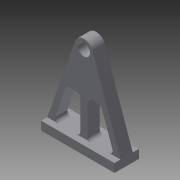
# Autodesk Inventor part: Y_axis_shaft_end_support
Saved by Autodesk Inventor 2013 (Build 170138000, 138)
## iProperties
Created: 2013-09-20
Part Number: Y_axis_shaft_end_support
Material: Aluminum 6061
Document SubType Name: Modeling
Designer: Ian
Density: 2.71 g/cm^3
Mass: 125.761 g
Surface Area: 152.318 cm^2
Volume: 46.4061 cm^3
d0: 3.500 in
d2: 0.500 in
d3: 0.750 in
d5: 1.500 in
d6: 90.00 deg
d7: 0.350 in
d14: 0.250 in
d16: 0.300 in
d17: 70.71 deg
d18: 0.150 in
d19: 0.300 in
d20: 0.300 in
d21: 0.300 in
d22: 0.150 in
d23: 0.150 in
d24: 0.500 in
d25: 0.150 in
d26: 0.500 in
d27: 0.00 deg
d28: 0.250 in
d29: 0.00 deg
Author: Ian
Autodesk Inventor part; units mm, degrees
ref_plane "YZ Plane" through (0, 0, 0) normal (1, 0, 0) x (0, 1, 0)
ref_plane "XZ Plane" through (0, 0, 0) normal (0, 1, 0) x (-1, 0, 0)
ref_plane "XY Plane" through (0, 0, 0) normal (0, 0, 1) x (1, 0, 0)
sketch "Sketch1" plane through (0, 0, 0) normal (0, 0, 1) x (1, 0, 0)
  line L0 (0, 0) -> (0, 88.9) construction
  circle A0 centre (0, 88.9) radius 6.35
  arc A1 (8.9901, 92.0471) -> (-8.9901, 92.0471) centre (0, 88.9) ccw
  line L1 (0, 0) -> (-38.1, 0)
  line L2 (-38.1, 0) -> (-38.1, 8.89)
  line L3 (-38.1, 8.89) -> (-8.9901, 92.0471)
  line L4 (0, 0) -> (38.1, 0)
  line L5 (38.1, 0) -> (38.1, 8.89)
  line L6 (38.1, 8.89) -> (8.9901, 92.0471)
  line L7 (-20.9396, 38.6924) -> (-28.6314, 16.7194)
  line L8 (-20.9396, 12.7) -> (0, 12.7) construction
  arc A2 (-29.5978, 13.9588) -> (-26.0017, 8.89) centre (-26.0017, 12.7) ccw
  line L9 (-28.6314, 16.7194) -> (-29.5978, 13.9588)
  line L10 (-20.9396, 8.89) -> (-26.0017, 8.89)
  line L11 (-20.9396, 12.7) -> (-26.0017, 12.7) construction
  circle A3 centre (0, 12.7) radius 3.81 construction
  arc A4 (-7.62, 8.89) -> (-3.81, 12.7) centre (-7.62, 12.7) ccw
  line L12 (-3.81, 12.7) -> (-3.81, 43.5601)
  line L13 (-26.0017, 12.7) -> (-13.8789, 47.3309) construction
  line L14 (-23.545, 50.4685) -> (0, 42.2264) construction
  line L15 (-24.8039, 46.8725) -> (0, 38.1897) construction
  line L16 (-20.9396, 38.6924) -> (-18.8105, 44.7745)
  line L17 (-15.2144, 43.5156) -> (-3.81, 43.5601) construction
  circle A5 centre (-3.81, 43.5601) radius 3.81 construction
  line L18 (-7.6348, 47.3552) -> (-15.2293, 47.3256)
  arc A6 (-15.2293, 47.3256) -> (-18.8105, 44.7745) centre (-15.2144, 43.5156) ccw
  arc A7 (-3.81, 43.5304) -> (-7.6348, 47.3552) centre (-7.62, 43.5452) ccw
  line L19 (-20.9396, 8.89) -> (-7.62, 8.89)
  line L20 (20.9396, 38.6924) -> (28.6314, 16.7194)
  arc A8 (26.0017, 8.89) -> (29.5978, 13.9588) centre (26.0017, 12.7) ccw
  line L21 (20.9396, 8.89) -> (26.0017, 8.89)
  arc A9 (3.81, 12.7) -> (7.62, 8.89) centre (7.62, 12.7) ccw
  line L22 (3.81, 12.7) -> (3.81, 43.5601)
  line L23 (20.9396, 38.6924) -> (18.8105, 44.7745)
  line L24 (7.6348, 47.3552) -> (15.2293, 47.3256)
  arc A10 (18.8105, 44.7745) -> (15.2293, 47.3256) centre (15.2144, 43.5156) ccw
  arc A11 (7.6348, 47.3552) -> (3.81, 43.5304) centre (7.62, 43.5452) ccw
  line L25 (20.9396, 8.89) -> (7.62, 8.89)
  line L26 (28.6314, 16.7194) -> (29.5978, 13.9588)
  point P0 (-3.81, 64.5628)
  dimension "d20" = 7.62
  dimension "d0" = 88.9
  dimension "d2" = 12.7
  dimension "d3" = 19.05
  dimension "d5" = 38.1
  dimension "d6" = 90
  dimension "d7" = 8.89
  dimension "d14" = 6.35
  dimension "d16" = 7.62
  dimension "d17" = 70.707
  dimension "d18" = 3.81
  dimension "d22" = 3.81
  dimension "d23" = 3.81
  dimension "d24" = 12.7
  dimension "d25" = 3.81
  constraints: 54 end point, 19 symmetric about line, 18 point on circle, 14 point on line, 10 centre point, 10 tangent, 5 coincident, 4 perpendicular, 3 parallel, 1 collinear, 1 horizontal, 1 horizontal alignment, 1 midpoint, 1 vertical, 9 other
  measures "d0" distance of L0.start L0.end
  measures "d2" diameter of A0
  measures "d3" diameter of A1
  measures "d5" distance of L0.start L1.end
  measures "d6" angle of L0 L1
  measures "d7" distance of L1.end L2.end
  measures "d14" distance between parallel lines of L7 L3
  measures "d16" diameter of A2
  measures "d17" angle of L8 L13
  measures "d18" distance between parallel lines of L14 L15
  measures "d22" radius of A6
  measures "d23" radius of A7
  measures "d24" distance from line of L1 L12.start
  measures "d25" radius of A4
extrude "Extrusion1" add sketch "Sketch1" along normal mid plane 12.7
sketch "Sketch2" plane through (0, 0, 6.35) normal (0, 0, 1) x (1, 0, 0)
  arc A0 (26.0017, 8.89) -> (29.5978, 13.9588) centre (26.0017, 12.7) ccw projected
  line L0 (26.0017, 8.89) -> (7.62, 8.89) projected
  arc A1 (3.81, 12.7) -> (7.62, 8.89) centre (7.62, 12.7) ccw projected
  line L1 (3.81, 12.7) -> (3.81, 43.5304) projected
  arc A2 (7.6348, 47.3552) -> (3.81, 43.5304) centre (7.62, 43.5452) ccw projected
  line L2 (7.6348, 47.3552) -> (15.2293, 47.3256) projected
  arc A3 (18.8105, 44.7745) -> (15.2293, 47.3256) centre (15.2144, 43.5156) ccw projected
  line L3 (18.8105, 44.7745) -> (29.5978, 13.9588) projected
  arc A4 (-15.2293, 47.3256) -> (-18.8105, 44.7745) centre (-15.2144, 43.5156) ccw projected
  line L4 (-15.2293, 47.3256) -> (-7.6348, 47.3552) projected
  arc A5 (-3.81, 43.5304) -> (-7.6348, 47.3552) centre (-7.62, 43.5452) ccw projected
  line L5 (-3.81, 43.5304) -> (-3.81, 12.7) projected
  arc A6 (-7.62, 8.89) -> (-3.81, 12.7) centre (-7.62, 12.7) ccw projected
  line L6 (-7.62, 8.89) -> (-26.0017, 8.89) projected
  arc A7 (-29.5978, 13.9588) -> (-26.0017, 8.89) centre (-26.0017, 12.7) ccw projected
  line L7 (-29.5978, 13.9588) -> (-18.8105, 44.7745) projected
  circle A8 centre (0, 88.9) radius 6.35 projected
  line L8 (-38.1, 0) -> (38.1, 0) projected
  line L9 (38.1, 0) -> (38.1, 8.89) projected
  line L10 (38.1, 8.89) -> (8.9901, 92.0471) projected
  arc A9 (8.9901, 92.0471) -> (-8.9901, 92.0471) centre (0, 88.9) ccw projected
  line L11 (-8.9901, 92.0471) -> (-38.1, 8.89) projected
  line L12 (-38.1, 8.89) -> (-38.1, 0) projected
  point P0 (0, 0)
sketch "Sketch3" plane through (0, 0, 6.35) normal (0, 0, 1) x (1, 0, 0)
  line L0 (-38.1, 0) -> (38.1, 0) projected
  line L1 (38.1, 0) -> (38.1, 8.89) projected
  line L2 (-38.1, 0) -> (38.1, 0)
  line L3 (38.1, 0) -> (38.1, 8.89)
  line L4 (38.1, 8.89) -> (-38.1, 8.89)
  line L5 (-38.1, 8.89) -> (-38.1, 0)
  point P0 (0, 0)
  constraints: 8 end point, 2 parallel, 1 horizontal, 1 perpendicular
extrude "Extrusion2" add sketch "Sketch3" along normal blind 6.35
mirror "Mirror1" about plane through (0, 0, 0) normal (0, 0, 1) of "Extrusion2"
body "Solid1"
